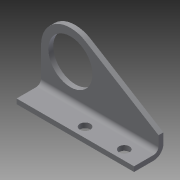
# Autodesk Inventor part: Flange Bearing Mount Tower
Saved by Autodesk Inventor 2013 (Build 170138000, 138)
## iProperties
Created: 2013-01-21
Part Number: Flange Bearing Mount Tower
Material: Generic
Document SubType Name: Sheet Metal
Designer: actoennies
Density: 1 g/cm^3
Sheet Metal Rule: Default
Mass: 13.7818 g
Surface Area: 100.387 cm^2
Volume: 13.7818 cm^3
Author: actoennies
Autodesk Inventor part; units mm, degrees
ref_plane "YZ Plane" through (0, 0, 0) normal (1, 0, 0) x (0, 1, 0)
ref_plane "XZ Plane" through (0, 0, 0) normal (0, 1, 0) x (-1, 0, 0)
ref_plane "XY Plane" through (0, 0, 0) normal (0, 0, 1) x (1, 0, 0)
sketch "Sketch1" plane through (0, 0, 0) normal (0, 1, 0) x (-1, 0, 0)
  line L0 (0, 0) -> (-101.6, 0)
  line L1 (-101.6, 0) -> (-101.6, 19.05)
  line L2 (0, 19.05) -> (0, 0)
  line L3 (0, 0) -> (-12.7, 0)
  circle A0 centre (-38.1, 12.7) radius 3.3782
  circle A1 centre (-63.5, 12.7) radius 3.3782
  line L4 (-101.6, 19.05) -> (0, 19.05)
  dimension "d2" = 101.6
  dimension "d5" = 6.7564
  dimension "d7" = 6.7564
  dimension "d9" = 38.1
  dimension "d57" = 19.05
  dimension "d58" = 6.35
  dimension "d59" = 6.35
  dimension "d60" = 25.4
  measures "d2" distance of L1.end L2.start
  measures "d5" diameter of A0
  measures "d7" diameter of A1
  measures "d9" distance from line of L2 A0.centre
  measures "d57" distance between parallel lines of L0 L4
  measures "d58" distance from line of L4 A1.centre
  measures "d59" distance from line of L4 A0.centre
  measures "d60" distance of A1.centre A0.centre
extrude "Plate2" add sketch "Sketch1" along normal blind 3.175
sketch "Sketch5" plane through (0, 4.445, -1.27) normal (0, 0, -1) x (-1, 0, 0)
  line L0 (-101.6, 0) -> (0, 0)
  line L1 (0, 0) -> (0, 40.005)
  line L2 (0, 40.005) -> (-101.6, 40.005)
  line L3 (-101.6, 40.005) -> (-101.6, 0)
  constraints: 6 end point, 1 horizontal, 1 perpendicular, 1 vertical
edge flange "Flange2" height 44.45 angle 90 thickness 3.175 bend radius 1.27 thickness toward (0, 0, -1) relief straight relief width 3.175 relief depth 1.5875 edges at (50.8, 3.175, 0) wall of the first edge with corners at (101.6, 4.445, -1.27) (0, 4.445, -1.27) (0, 44.45, -1.27) (101.6, 44.45, -1.27)
bend "Bend2"
corner "Corner2"
sketch "Sketch6" plane through (0, 44.45, -1.27) normal (0, 0, 1) x (1, 0, 0)
  line L0 (0, -40.005) -> (101.6, -40.005) projected
  line L1 (101.6, 0) -> (101.6, -40.005) projected
  line L2 (101.6, 0) -> (0, 0) projected
  line L3 (0, 0) -> (0, -40.005) projected
  circle A0 centre (19.05, -19.05) radius 14.2875
  arc A1 (26.5447, -1.5363) -> (0, -19.05) centre (19.05, -19.05) ccw
  line L4 (101.6, -33.655) -> (26.5447, -1.5363)
  point P0 (0, -44.45)
  dimension "d50" = 28.575
  dimension "d51" = 19.05
  dimension "d52" = 19.05
  dimension "d53" = 6.35
  constraints: 2 centre point, 2 end point, 2 point on circle, 2 point on line, 2 tangent, 1 coincident
  measures "d50" diameter of A0
  measures "d51" distance from line of L2 A0.centre
  measures "d52" distance from line of L3 A0.centre
  measures "d53" distance of L0.end L4.start
extrude "Cut3" cut sketch "Sketch6" against normal blind 3.175 contours L3 L2 A1 | L4 A1 L2 L1 | A0
equation "\"d54\" = Thickness"
equation "\"d40\" = BendReliefWidth"
equation "\"d41\" = BendReliefDepth"
equation "\"d42\" = MinimumRemnant"
equation "\"d43\" = BendRadius"
equation "\"d47\" = CornerReliefSize"
equation "\"d48\" = GapSize"
equation "\"d49\" = JacobiRadiusSize"
equation "\"BendRadius\" = Thickness"
equation "\"BendReliefWidth\" = Thickness"
equation "\"BendReliefDepth\" = 0.5 * Thickness"
equation "\"CornerReliefSize\" = 4 * Thickness"
equation "\"MinimumRemnant\" = 2 * Thickness"
equation "\"TransitionRadius\" = BendRadius"
equation "\"JacobiRadiusSize\" = BendRadius"
equation "\"GapSize\" = Thickness"
equation "\"d18\" = BendRadius"
equation "\"d19\" = BendRadius"
equation "\"Thickness\" = 3.175"
body "Solid2"
